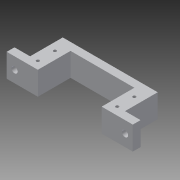
# Autodesk Inventor part: PinewoodServoMount
Saved by Autodesk Inventor 2013 (Build 170138000, 138)
## iProperties
Created: 2015-05-14
Part Number: PinewoodServoMount
Material: Generic
Document SubType Name: Modeling
Designer: joshgunnar
Density: 1 g/cm^3
Author: joshgunnar
Autodesk Inventor part; units mm, degrees
ref_plane "YZ Plane" through (0, 0, 0) normal (1, 0, 0) x (0, 1, 0)
ref_plane "XZ Plane" through (0, 0, 0) normal (0, 1, 0) x (-1, 0, 0)
ref_plane "XY Plane" through (0, 0, 0) normal (0, 0, 1) x (1, 0, 0)
sketch "Sketch1" plane through (0, 0, 0) normal (0, 0, 1) x (1, 0, 0)
  line L0 (-20.5, -10.5) -> (20.5, -10.5)
  line L1 (20.5, -10.5) -> (20.5, 10.5)
  line L2 (20.5, 10.5) -> (-20.5, 10.5)
  line L3 (-20.5, 10.5) -> (-20.5, -10.5)
  line L4 (-20.5, -10.5) -> (20.5, 10.5) construction
  line L5 (20.5, -10.5) -> (-20.5, 10.5) construction
  circle A0 centre (25.5, 5.5) radius 1
  circle A1 centre (25.5, -5.5) radius 1
  line L6 (0, 21.6766) -> (0, -21.497) construction
  circle A2 centre (-25.5, 5.5) radius 1
  circle A3 centre (-25.5, -5.5) radius 1
  line L7 (-20.5, -10.5) -> (-30.5, -10.5)
  line L8 (-30.5, -10.5) -> (-30.5, 10.5)
  line L9 (-30.5, 10.5) -> (-20.5, 10.5)
  line L10 (-20.5, 10.5) -> (-20.5, -10.5)
  line L11 (20.5, -10.5) -> (30.5, -10.5)
  line L12 (30.5, -10.5) -> (30.5, 10.5)
  line L13 (30.5, 10.5) -> (20.5, 10.5)
  line L14 (20.5, 10.5) -> (20.5, -10.5)
  line L15 (-30.5, 10.5) -> (30.5, 10.5)
  line L16 (30.5, 10.5) -> (30.5, 15.5)
  line L17 (30.5, 15.5) -> (-30.5, 15.5)
  line L18 (-30.5, 15.5) -> (-30.5, 10.5)
  line L19 (-30.5, -10.5) -> (-40.5, -10.5)
  line L20 (-40.5, -10.5) -> (-40.5, -5.5)
  line L21 (-40.5, -5.5) -> (-30.5, -5.5)
  line L22 (-30.5, -5.5) -> (-30.5, -10.5)
  line L23 (30.5, -10.5) -> (40.5, -10.5)
  line L24 (40.5, -10.5) -> (40.5, -5.5)
  line L25 (40.5, -5.5) -> (30.5, -5.5)
  line L26 (30.5, -5.5) -> (30.5, -10.5)
  point P0 (0, 0)
  dimension "d0" = 41
  dimension "d1" = 21
  dimension "d2" = 2
  dimension "d3" = 2
  dimension "d4" = 10
  dimension "d5" = 10
  dimension "d6" = 5
  dimension "d7" = 10
  dimension "d8" = 5
  dimension "d9" = 10
  constraints: 54 end point, 13 parallel, 6 horizontal, 6 perpendicular, 4 centre point, 2 midpoint, 2 symmetric about line, 2 other
  measures "d0" distance of L0.start L0.end
  measures "d1" distance of L1.end L0.end
  measures "d2" diameter of A0
  measures "d3" diameter of A1
  measures "d4" distance of L8.end L9.end
  measures "d5" distance of L13.end L12.end
  measures "d6" distance of L16.end L15.end
  measures "d7" distance of L20.end L21.end
  measures "d8" distance of L19.end L20.end
  measures "d9" distance of L25.end L24.end
extrude "Extrusion1" add sketch "Sketch1" along normal blind 15 contours L7 L8 L9 L3 | L1 L13 L12 L11 | L9 L18 L17 L16 L13 L2 | L19 L20 L21 L8 | L12 L25 L24 L23
sketch "Sketch2" plane through (30.5, -5.5, 0) normal (0, 1, 0) x (1, 0, 0)
  circle A0 centre (5, -7.5) radius 2
  point P0 (-30.5, 0)
  dimension "d12" = 4
  constraints: 1 centre point
  measures "d12" diameter of A0
extrude "Extrusion2" cut sketch "Sketch2" against normal through all
mirror "Mirror1" about plane through (0, 0, 0) normal (1, 0, 0) of "Extrusion2"
body "Solid1"
